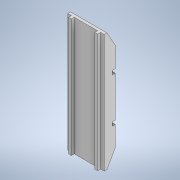
# Autodesk Inventor part: X_axis
Saved by Autodesk Inventor 2020 (Build 240168000, 168)
## iProperties
Created: 2020-05-02
Part Number: X_axis
Material: Generic
Document SubType Name: Modeling
Designer: zhang
Density: 1 g/cm^3
Appearance: Default
Author: zhang
Autodesk Inventor part; units mm, degrees
ref_plane "YZ Plane" through (0, 0, 0) normal (1, 0, 0) x (0, 1, 0)
ref_plane "XZ Plane" through (0, 0, 0) normal (0, 1, 0) x (-1, 0, 0)
ref_plane "XY Plane" through (0, 0, 0) normal (0, 0, 1) x (1, 0, 0)
sketch "Sketch1" plane through (0, 0, 0) normal (0, 1, 0) x (-1, 0, 0)
  line L0 (100, -195) -> (-100, -195)
  line L1 (-100, -195) -> (-100, -255)
  line L2 (-100, -255) -> (100, -255)
  line L3 (100, -255) -> (100, -195)
  line L4 (0, 66.9735) -> (0, -172.2265)
  point P0 (0, 0)
  dimension "d0" = 200
  dimension "d1" = 60
  dimension "d2" = 195
  constraints: 10 end point, 2 parallel, 2 vertical, 1 horizontal, 1 perpendicular, 1 other
  measures "d0" distance of L0.start L0.end
  measures "d1" distance of L0.end L1.end
  measures "d2" distance from line of L0 point (0, 0)
extrude "Extrusion1" add sketch "Sketch1" along normal mid plane 650
chamfer "Chamfer1" distance 45 distance2 80 1 edges at (0, 325, -255) measured on face at (33.3333, 325, -215)
chamfer "Chamfer2" distance 45 distance2 80 1 edges at (0, -325, -255) measured on face at (33.3333, -325, -215)
sketch "Sketch2" plane through (0, -325, 0) normal (0, -1, 0) x (1, 0, 0)
  line L0 (100, -195) -> (-100, -195) projected
  line L1 (-80, -179) -> (-64, -179)
  line L2 (-64, -179) -> (-64, -195)
  line L3 (-64, -195) -> (-80, -195)
  line L4 (-80, -195) -> (-80, -179)
  line L5 (-100, -195) -> (-100, -210) projected
  line L6 (0, 0) -> (0, -427.5887)
  line L7 (80, -179) -> (64, -179)
  line L8 (64, -179) -> (64, -195)
  line L9 (64, -195) -> (80, -195)
  line L10 (80, -195) -> (80, -179)
  dimension "d11" = 20
  dimension "d12" = 16
  dimension "d13" = 16
  constraints: 18 end point, 4 symmetric about line, 2 parallel, 1 horizontal, 1 perpendicular, 1 point on line, 1 vertical
  measures "d11" distance between parallel lines of L5 L4
  measures "d12" distance of L1.start L1.end
  measures "d13" distance of L1.end L2.end
extrude "Extrusion2" add sketch "Sketch2" against normal blind 650
sketch "Sketch3" plane through (100, -325, -195) normal (1, 0, 0) x (0, 0, -1)
  line L0 (-195, 325) -> (152.733, 325)
  line L1 (60, 80) -> (60, 570) projected
  line L2 (60, 193) -> (44, 193)
  line L3 (44, 193) -> (44, 213)
  line L4 (44, 213) -> (60, 213)
  line L5 (60, 213) -> (60, 193)
  line L6 (60, 457) -> (44, 457)
  line L7 (44, 457) -> (44, 437)
  line L8 (44, 437) -> (60, 437)
  line L9 (60, 437) -> (60, 457)
  point P0 (60, 437)
  point P1 (60, 213)
  dimension "d16" = 224
  dimension "d17" = 16
  dimension "d18" = 20
  constraints: 18 end point, 4 symmetric about line, 2 horizontal, 2 parallel, 1 perpendicular, 1 point on line
  measures "d16" diameter of L4 L0
  measures "d17" distance of L3.end L4.end
  measures "d18" distance of L2.end L3.end
extrude "Extrusion3" cut sketch "Sketch3" against normal through all
body "Solid1"
